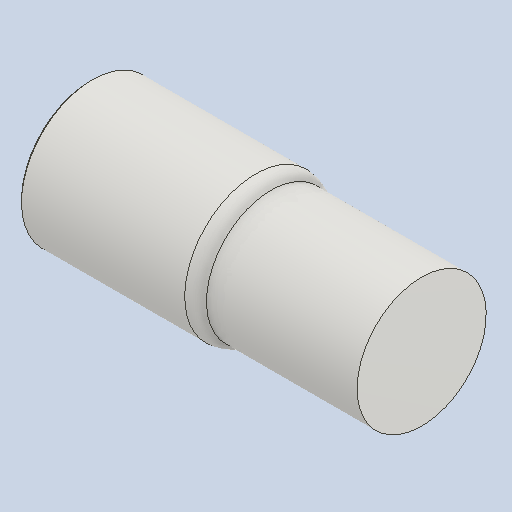
# Autodesk Inventor part: Shaft
Saved by Autodesk Inventor 2023 (Build 270158000, 158)
## iProperties
Created: 2023-01-29
Part Number: Shaft
Material: Steel
Document SubType Name: Modeling
Designer: Merve Babacan
Density: 1 g/cm^3
Appearance: Steel
CustomPartVersion: 1
Author: Merve Babacan
Length: 77.000 mm
Autodesk Inventor part; units mm, degrees
ref_plane "Start Plane" through (0, 0, 0) normal (1, 0, 0) x (0, 1, 0)
ref_plane "XZ Plane" through (0, 0, 0) normal (0, 1, 0) x (-1, 0, 0)
ref_plane "XY Plane" through (0, 0, 0) normal (0, 0, 1) x (1, 0, 0)
sketch "Main Sketch" plane through (0, 0, 0) normal (0, 0, 1) x (1, 0, 0)
  line L0 (0, 0) -> (77, 0)
  line L1 (0, 0) -> (0, 16.5)
  line L2 (42, 16.5) -> (42, 15)
  line L3 (0, 16.5) -> (42, 16.5)
  line L4 (77, 15) -> (77, 0)
  line L5 (42, 15) -> (77, 15)
  dimension "d3" = 33
  dimension "d4" = 30
  constraints: 12 end point, 4 horizontal, 3 vertical
  measures "d3" diameter of L3 L0
  measures "d4" diameter of L5 L0
revolve "Revolution1" add sketch "Main Sketch" angle 360 about axis through (0, 0, 0) along (1, 0, 0)
chamfer "Chamfer1" distance 0.5 angle 45 1 edges at (0, -16.5, 0) measured on face at (28, 16.4465, -1.3277)
fillet "Fillet1" radius 5 1 edges at (42, -16.5, 0)
equation "\"Length\" = 77"
body "Solid1"
